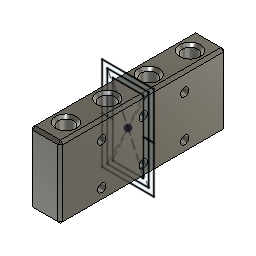
Crush Block (Parametric) (Autodesk Fusion 360 design; units mm, degrees)
Autodesk Fusion 360 part; units mm, degrees
sketch "Sketch1" plane through (0, 0, 0) normal (0, 1, 0) x (1, 0, 0)
  line L0 (9.3345, 22.0345) -> (-9.3345, 22.0345)
  line L1 (-9.3345, 22.0345) -> (-9.3345, -22.0345)
  line L2 (-9.3345, -22.0345) -> (9.3345, -22.0345)
  line L3 (9.3345, -22.0345) -> (9.3345, 22.0345)
  line L4 (9.3345, 22.0345) -> (-9.3345, -22.0345) construction
  line L5 (-9.3345, 22.0345) -> (9.3345, -22.0345) construction
  line L6 (12.7, -25.4) -> (-12.7, -25.4)
  line L7 (-12.7, -25.4) -> (-12.7, 25.4)
  line L8 (-12.7, 25.4) -> (12.7, 25.4)
  line L9 (12.7, 25.4) -> (12.7, -25.4)
  line L10 (12.7, -25.4) -> (-12.7, 25.4) construction
  line L11 (-12.7, -25.4) -> (12.7, 25.4) construction
  line L12 (-9.3345, 0) -> (-12.7, 0)
  line L13 (9.3345, 0) -> (12.7, 0)
  line L14 (-15.875, -28.575) -> (-15.875, 28.575)
  line L15 (-15.875, 28.575) -> (15.875, 28.575)
  line L16 (15.875, 28.575) -> (15.875, -28.575)
  line L17 (15.875, -28.575) -> (-15.875, -28.575)
  line L18 (12.7, 0) -> (15.875, 0)
  line L19 (-12.7, 0) -> (-15.875, 0)
  dimension "d32" = 25.4
  dimension "d33" = 50.8
  dimension "d34" = 3.3655
  dimension "d35" = 3.3655
  dimension "d43" = -3.175
  constraint horizontal L0
  constraint perpendicular L0 L1
  constraint parallel L0 L2
  constraint parallel L1 L3
  constraint coincident L4 origin
  constraint coincident L5 origin
  constraint horizontal L6
  constraint perpendicular L6 L7
  constraint parallel L6 L8
  constraint parallel L7 L9
  constraint coincident L10 origin
  constraint coincident L11 origin
  constraint midpoint L1 L12.start
  constraint midpoint L7 L12.end
  constraint midpoint L3 L13.start
  constraint midpoint L9 L13.end
  constraint midpoint L16 L18.end
  constraint midpoint L14 L19.end
  measures "d32" distance of L7.end L8.end
  measures "d33" distance of L6.end L7.end
  measures "d34" distance of L2 L6
  measures "d35" distance of L1 L7
extrude "Extrude1" add sketch "Sketch1" along normal mid plane 101.6 contours L0 L1 L2 L3 makes body 1
sketch "Sketch2" plane through (0, 0, 22.0345) normal (0, 0, 1) x (-1, 0, 0)
  line L0 (-9.3345, 50.8) -> (-9.3345, -50.8) construction
  line L1 (-9.3345, -50.8) -> (9.3345, -50.8) construction
  line L2 (9.3345, -50.8) -> (9.3345, 50.8) construction
  line L3 (9.3345, 50.8) -> (-9.3345, 50.8) construction
  line L4 (0, 50.8) -> (0, -50.8) construction
  circle A0 centre (0, 38.1) radius 4.7625
  line L5 (0, 25.4) -> (0, -76.2) construction
  line L6 (0, 0) -> (0, -101.6) construction
  line L7 (0, -25.4) -> (0, -127) construction
  dimension "d9" = 9.525
  constraint midpoint L3 L4.start
  constraint midpoint L1 L4.end
  constraint coincident L4 A0.centre
  measures "d9" diameter of A0
extrude "Extrude2" cut sketch "Sketch2" against normal through all bodies 1
pattern_linear "R-Pattern1" count 4 spacing 25.4 along (0, 1, 0) of "Extrude2"
sketch "Sketch3" plane through (9.3345, 0, 0) normal (1, 0, 0) x (0, 1, 0)
  line L0 (-50.8, -22.0345) -> (50.8, -22.0345) construction
  line L1 (50.8, -22.0345) -> (50.8, 22.0345) construction
  line L2 (50.8, 22.0345) -> (-50.8, 22.0345) construction
  line L3 (-50.8, 22.0345) -> (-50.8, -22.0345) construction
  line L4 (0, 22.0345) -> (0, -22.0345) construction
  line L5 (-50.8, 0) -> (50.8, 0) construction
  circle A0 centre (-25.4, 11.0172) radius 2.54
  circle A1 centre (-25.4, 11.0172) radius 4.7625
  line L6 (-50.8, 11.0172) -> (50.8, 11.0172) construction
  dimension "d16" = 5.08
  dimension "d17" = 9.525
  dimension "d18" = 25.4
  constraint midpoint L3 L5.start
  constraint midpoint L1 L5.end
  constraint concentric A0 A1
  constraint coincident L3 L6.start
  constraint coincident L1 L6.end
  constraint perpendicular L1 L6
  constraint symmetric L2 L5 L6
  constraint coincident A0.centre L6
  measures "d16" diameter of A0
  measures "d17" diameter of A1
  measures "d18" distance of L3 A0.centre
extrude "Extrude3" cut sketch "Sketch3" against normal through all contours A0 bodies 1
extrude "Extrude4" cut sketch "Sketch3" against normal up to surface (5.969 mm away) from surface at -6.35 bodies 1
pattern_linear "R-Pattern2" count 3 spacing 25.4 along (0, 1, 0) count 2 spacing 25.4 along (0, 0, -1) of "Extrude3", "Extrude4"
chamfer "Chamfer1" distance 1.5875 angle 45 4 faces at (-0.1186, 48.1497, 22.0345) (3.1115, -50.8, -7.3448) (0.1186, 48.1497, -22.0345) (3.1115, 50.8, -7.3448) on bodies 1
extrude "Extrude1'" add sketch "Sketch1" along normal mid plane 38.1 separate body contours L6 L7 L9 L14 L16 L17 L18 L19 makes body 2 in component "Drill Guide"
sketch "Sketch1 (2)" plane through (0, 0, 25.4) normal (0, 0, -1) x (-1, 0, 0) in component "Drill Guide"
  line L0 (-12.7, 19.05) -> (-12.7, -19.05)
  line L1 (12.7, 19.05) -> (-12.7, 19.05)
  line L2 (12.7, -19.05) -> (12.7, 19.05)
  line L3 (-12.7, -19.05) -> (12.7, -19.05)
  circle A0 centre (0, 12.7) radius 6.35 construction
  circle A1 centre (0, -12.7) radius 6.35 construction
hole "Hole1" at (0, -12.7, 25.4) at (0, 12.7, 25.4) direction (0, 0, 1) diameter 6.5278 end through all bodies 2 in component "Drill Guide"
sketch "Sketch2 (2)" plane through (12.7, 0, 0) normal (-1, 0, 0) x (0, 1, 0) in component "Drill Guide"
  line L0 (19.05, -25.4) -> (19.05, 0)
  line L1 (-19.05, -25.4) -> (19.05, -25.4)
  line L2 (-19.05, 0) -> (-19.05, -25.4)
  circle A0 centre (0, -11.0172) radius 2.54 construction
  circle A1 centre (0, -11.0172) radius 2.54
  line L3 (19.05, 0) -> (-19.05, 0)
extrude "Extrude2'" cut sketch "Sketch2 (2)" against normal through all contours A1 bodies 2 in component "Drill Guide"
chamfer "Chamfer1'" distance 12.7 angle 45 4 edges at (14.2875, -19.05, 0) (-14.2875, -19.05, 0) (-14.2875, 19.05, 0) (14.2875, 19.05, 0) on bodies 2 in component "Drill Guide"
component "Drill Guide" placed x (1, 0, 0) y (0, 1, 0) z (0, 0, 1) at (0, 0, 0)
equation "WIDTH = 1 in"
equation "HEIGHT = 2 in"
equation "LENGTH = 4 in"
equation "WALL = 0.125 in" comment "Wall thickness (nominal)"
equation "d7 = LENGTH"
equation "d19 = LENGTH / 1 in"
equation "d27 = ( LENGTH / 1 in ) - 1"
equation "d32 = WIDTH"
equation "d33 = HEIGHT"
equation "d34 = WALL + TOLERANCE / 2"
equation "d35 = WALL + TOLERANCE / 2"
equation "TOLERANCE = 0.015 in" comment "Tolerance on width, height axis"
named bodies: "Block"
